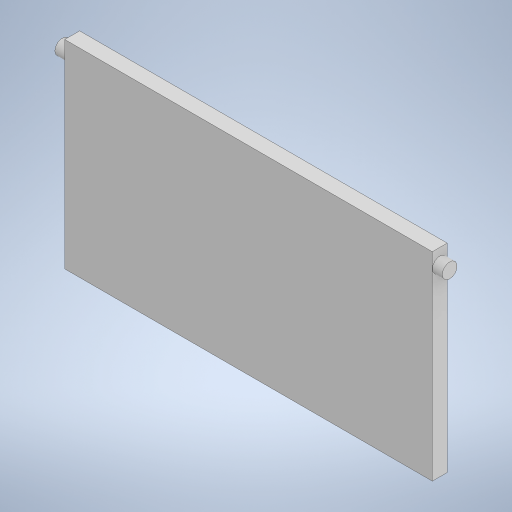
# Autodesk Inventor part: 挡板
Saved by Autodesk Inventor 2023.1 (Build 271208000, 208)
## iProperties
Created: 2023-07-19
Part Number: 挡板
Material: 常规
Document SubType Name: Modeling
Designer: Selcon
Density: 1 g/cm^3
Appearance: 默认
Author: Selcon
Autodesk Inventor part; units mm, degrees
ref_plane "YZ Plane" through (0, 0, 0) normal (1, 0, 0) x (0, 1, 0)
ref_plane "XZ Plane" through (0, 0, 0) normal (0, 1, 0) x (-1, 0, 0)
ref_plane "XY Plane" through (0, 0, 0) normal (0, 0, 1) x (1, 0, 0)
sketch "草图1" plane through (0, 0, 0) normal (1, 0, 0) x (0, 1, 0)
  line L0 (100, 7.5) -> (-100, 7.5)
  line L1 (-100, 7.5) -> (-100, -7.5)
  line L2 (-100, -7.5) -> (100, -7.5)
  line L3 (100, -7.5) -> (100, 7.5)
  line L4 (0, -10.5) -> (0, 10.5) projected
  line L5 (-140, 0) -> (140, 0) projected
  point P0 (0, 0)
  dimension "d0" = 15
  dimension "d1" = 200
  constraints: 8 end point, 2 parallel, 1 horizontal, 1 perpendicular, 2 other
  measures "d0" distance of L2.end L0.start
  measures "d1" distance of L1.end L2.end
extrude "拉伸1" add sketch "草图1" along normal mid plane 370
sketch "草图2" plane through (-185, 0, 0) normal (-1, 0, 0) x (0, 0, 1)
  line L0 (0, -148.5) -> (0, 191) projected
  circle A0 centre (0, 85) radius 7.5
  line L1 (7.5, 100) -> (-7.5, 100) projected
  point P0 (0, 0)
  dimension "d4" = 15
  dimension "d5" = 15
  constraints: 1 centre point, 1 point on line
  measures "d4" diameter of A0
  measures "d5" distance from line of L1 A0.centre
extrude "拉伸2" add sketch "草图2" along normal blind 10
mirror "镜像1" about plane through (0, 0, 0) normal (1, 0, 0) of "拉伸2"
